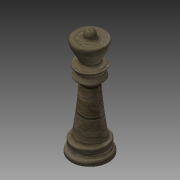
# Autodesk Inventor part: Queen
Saved by Autodesk Inventor 2015 SP1 (Build 190203100, 203)
## iProperties
Created: 2015-06-07
Part Number: Queen
Material: Wood (Cherry)
Document SubType Name: Modeling
Designer: Nathan
Density: 0.63 g/cm^3
Appearance: Driftwood
Author: Nathan
Autodesk Inventor part; units mm, degrees
ref_plane "YZ Plane" through (0, 0, 0) normal (1, 0, 0) x (0, 1, 0)
ref_plane "XZ Plane" through (0, 0, 0) normal (0, 1, 0) x (-1, 0, 0)
ref_plane "XY Plane" through (0, 0, 0) normal (0, 0, 1) x (1, 0, 0)
sketch "Sketch1" plane through (0, 0, 0) normal (0, 0, 1) x (1, 0, 0)
  line L0 (0, 10.7167) -> (0, 0)
  line L1 (0, 0) -> (14.846, 0)
  arc A0 (12.9584, 6.4952) -> (13.7958, 3.4613) centre (14.831, 5.3796) ccw
  line L2 (13.2402, 9.7167) -> (13.2402, 7.5188)
  line L3 (14.846, 1.7013) -> (14.846, 0)
  arc A1 (12.9584, 6.4952) -> (13.2402, 7.5188) centre (11.2402, 7.5188) ccw
  arc A2 (14.846, 1.7013) -> (13.7958, 3.4613) centre (12.846, 1.7013) ccw
  arc A3 (13.2402, 9.7167) -> (12.2402, 10.7167) centre (12.2402, 9.7167) ccw
  line L4 (0, 0) -> (0, 10.7167)
  line L5 (12.2402, 10.7167) -> (10.8438, 10.7167)
  ellipse E0 centre (0, 81.2166) end of major axis (3.9001, 81.2166) minor radius 3.7834 (3.2339, 79.1018) -> (0, 85) ccw
  line L6 (3.2339, 79.1018) -> (6.5093, 77.8043)
  line L7 (11.4391, 73.4449) -> (5.3021, 62.1073)
  spline S0 degree 4 poles (5.3021, 62.1073) (6.1463, 61.627) (8.9371, 62.8381) (8.9849, 60.3944) (11.0597, 61.1543) (10.6135, 59.4753) knots 1.255588 1.255588 1.255588 1.255588 1.255588 2 2.137857 2.137857 2.137857 2.137857 2.137857
  arc A4 (11.4391, 73.4449) -> (11.6567, 74.091) centre (9.6803, 74.3969) ccw
  line L8 (10.6135, 59.4753) -> (7.9981, 56.7612) construction
  line L9 (7.9981, 56.7612) -> (8.8076, 55.8096) construction
  line L10 (8.8076, 55.8096) -> (9.2343, 54.6763) construction
  line L11 (9.2343, 54.6763) -> (11.3444, 52.1035) construction
  spline S1 degree 4 poles (10.6135, 59.4753) (7.9981, 56.7612) (8.8076, 55.8096) (9.2343, 54.6763) (11.3444, 52.1035) (9.0433, 52.4248) (7.6536, 51.3263) (6.5238, 50.4268) knots 1 1 1 1 1 2 3 4 4.74577 4.74577 4.74577 4.74577 4.74577
  line L12 (8.9849, 60.3944) -> (11.0597, 61.1543) construction
  line L13 (11.0597, 61.1543) -> (10.6135, 59.4753) construction
  line L14 (0, 85) -> (0, 0)
  line L15 (6.5093, 77.8043) -> (7.7716, 77.8043) construction
  line L16 (7.7716, 77.8043) -> (8.3549, 78.1518) construction
  line L17 (8.3549, 78.1518) -> (9.3077, 78.5013) construction
  line L18 (9.3077, 78.5013) -> (9.6803, 78.5013) construction
  line L19 (9.6803, 78.5013) -> (11.6567, 78.5013) construction
  line L20 (11.6567, 78.5013) -> (11.6567, 78.5013) construction
  line L21 (11.6567, 78.5013) -> (12.506, 77.0253) construction
  line L22 (12.506, 77.0253) -> (11.6567, 74.091) construction
  spline S2 degree 4 poles (6.5093, 77.8043) (7.7716, 77.8043) (8.3549, 78.1518) (9.3077, 78.5013) (9.6803, 78.5013) (11.6567, 78.5013) (11.6567, 78.5013) (12.506, 77.0253) (11.6567, 74.091) knots 1 1 1 1 1 2 3 4 5 6 6 6 6 6
  line L23 (10.8438, 10.7167) -> (10.1547, 12.2582) construction
  spline S3 degree 4 poles (10.8438, 10.7167) (10.1547, 12.2582) (8.9159, 22.7774) (6.7343, 35.3682) (6.5238, 50.4268) knots 1 1 1 1 1 1.967221 1.967221 1.967221 1.967221 1.967221
  line L24 (10.1547, 12.2582) -> (8.9159, 22.7774) construction
  line L25 (8.9159, 22.7774) -> (6.7343, 35.3682) construction
  line L26 (6.7343, 35.3682) -> (6.5238, 50.4268) construction
  line L27 (11.3444, 52.1035) -> (9.0433, 52.4248) construction
  line L28 (9.0433, 52.4248) -> (7.6536, 51.3263) construction
  line L29 (7.6536, 51.3263) -> (6.5238, 50.4268) construction
  line L30 (5.3021, 62.1073) -> (6.1463, 61.627) construction
  line L31 (6.1463, 61.627) -> (8.9371, 62.8381) construction
  line L32 (8.9371, 62.8381) -> (8.9849, 60.3944) construction
  line L33 (0, 0) -> (14.846, 0)
  line L34 (14.846, 0) -> (0, 0)
  line L35 (0, 0) -> (0, 85)
  point P0 (14.846, 3.1999)
  point P1 (13.2402, 6.8697)
  dimension "d11" = 2
  dimension "d13" = 1
  dimension "d35" = 2
  dimension "d39" = 85
  constraints: 24 end point, 13 point on circle, 7 tangent, 5 centre point, 5 horizontal, 3 vertical, 2 collinear, 2 point on line, 1 equal radius, 16 other
  measures "d11" radius of A1
  measures "d13" radius of A3
  measures "d35" radius of A4
  measures "d39" distance of L14.start L0.end
revolve "Revolution2" add sketch "Sketch1" angle 360 about axis through (0, 85, 0) along (0, -1, 0)
fillet "Fillet6" radius 2 5 edges at (-6.5238, 50.4268, 0) (-5.3021, 62.1073, 0) (-3.2339, 79.1018, 0) (-10.8438, 10.7167, 0) (-10.6135, 59.4753, 0)
body "Solid2"
